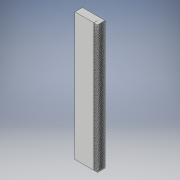
# Autodesk Inventor part: GearLiftProtoPart1
Saved by Autodesk Inventor 2017 (Build 210142000, 142)
## iProperties
Created: 2017-11-15
Part Number: GearLiftProtoPart1
Material: Generic
Document SubType Name: Modeling
Designer: User
Density: 1 g/cm^3
Appearance: Default
Author: User
Autodesk Inventor part; units mm, degrees
ref_plane "YZ Plane" through (0, 0, 0) normal (1, 0, 0) x (0, 1, 0)
ref_plane "XZ Plane" through (0, 0, 0) normal (0, 1, 0) x (-1, 0, 0)
ref_plane "XY Plane" through (0, 0, 0) normal (0, 0, 1) x (1, 0, 0)
sketch "Sketch1" plane through (0, 0, 0) normal (0, 0, 1) x (1, 0, 0)
  line L0 (0, 0) -> (-76.2, 0)
  line L1 (-76.2, 0) -> (-76.2, -431.8)
  line L2 (-76.2, -431.8) -> (0, -431.8)
  line L3 (0, -431.8) -> (0, 0)
  dimension "d0" = 76.2
  dimension "d1" = 431.8
  constraints: 8 end point, 2 parallel, 1 horizontal, 1 perpendicular
  measures "d0" distance of L2.end L1.end
  measures "d1" distance of L1.end L0.end
extrude "Extrusion1" add sketch "Sketch1" along normal blind 25.4
sketch "Sketch2" plane through (0, 0, 25.4) normal (0, 0, 1) x (1, 0, 0)
  line L0 (0, 0) -> (-76.2, 0) projected
  line L1 (0, 0) -> (-12.7, 0)
  line L2 (-12.7, 0) -> (-12.7, -431.8)
  line L3 (-76.2, -431.8) -> (0, -431.8) projected
  line L4 (0, -431.8) -> (0, 0) projected
  line L5 (0, -431.8) -> (0, 0)
  dimension "d4" = 12.7
  constraints: 6 end point, 2 point on line, 1 collinear, 1 perpendicular
  measures "d4" distance of L0.start L1.end
sketch "Sketch3" plane through (0, -431.8, 0) normal (1, 0, 0) x (0, 0, -1)
  line L0 (-25.4, 0) -> (-25.4, 431.8) projected
  line L1 (-25.4, 431.8) -> (0, 430.691)
  line L2 (0, 0) -> (0, 431.8) projected
  line L3 (-25.4, 431.8) -> (0.0242, 431.8) construction
  line L4 (0, 430.691) -> (-25.4, 429.582)
  line L5 (-25.4, 431.8) -> (-25.4, 0) projected
  dimension "d18" = 5
  dimension "d19" = 87.5
  constraints: 6 end point, 2 point on line, 1 equal length, 1 horizontal
  measures "d18" angle of L1 L4
  measures "d19" angle of L2 L1
extrude "Extrusion2" cut sketch "Sketch3" against normal blind 12.7
pattern_linear "Rectangular Pattern2" count 188 spacing 2.286 along (0, -1, 0) of "Extrusion2"
body "Solid1"
